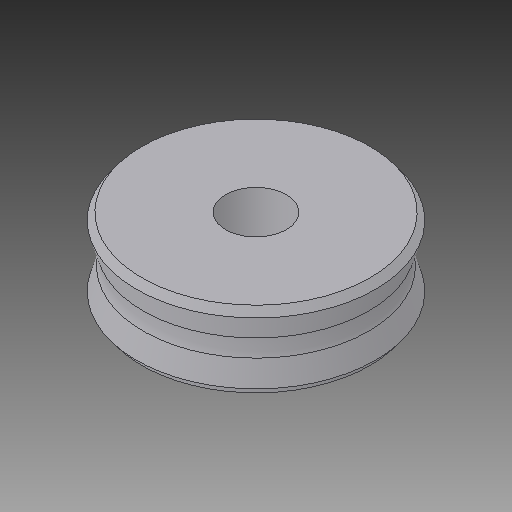
# Autodesk Inventor part: Roulement a bille 634ZZ
Saved by Autodesk Inventor 2017 (Build 210142000, 142)
## iProperties
Company: FABLAB Frenchmakers
Part Number: Roulement a bille 634ZZ
Material: ----------
Document SubType Name: Modeling
Designer: FABLAB Frenchmakers
Density: 7.86 g/cm^3
Appearance: Métal - Acier
Mass: 6.61052 g
Surface Area: 6.47649 cm^2
Volume: 0.841033 cm^3
Project: 1420 Vauban 3D XL
Catalog Web Link: http://frenchmakers.com/
Stock Number: 1420-05-17
Autodesk Inventor part; units mm, degrees
ref_plane "YZ Plane" through (0, 0, 0) normal (1, 0, 0) x (0, 1, 0)
ref_plane "XZ Plane" through (0, 0, 0) normal (0, 1, 0) x (-1, 0, 0)
ref_plane "XY Plane" through (0, 0, 0) normal (0, 0, 1) x (1, 0, 0)
sketch "Esquisse1" plane through (0, 0, 0) normal (0, 0, 1) x (1, 0, 0)
  line L0 (0, 0) -> (0, 2.5152)
  line L1 (2, -2.5) -> (2, 2.5)
  line L2 (2, 2.5) -> (8, 2.5)
  line L3 (8, 2.5) -> (7.4224, 0.5747)
  line L4 (7.4224, -0.5747) -> (8, -2.5)
  line L5 (8, -2.5) -> (2, -2.5)
  arc A0 (7.4224, 0.5747) -> (7.4224, -0.5747) centre (9.3381, 0) ccw
  point P0 (7.25, 0)
  dimension "d0" = 4
  dimension "d1" = 5
  dimension "d2" = 2.5
  dimension "d3" = 16
  dimension "d4" = 14.5
  dimension "d5" = 2
  constraints: 12 end point, 2 point on circle, 2 point on line, 2 tangent, 2 vertical, 1 centre point, 1 horizontal, 1 horizontal alignment, 1 parallel, 1 vertical alignment
  measures "d0" diameter of L1 L0
  measures "d1" distance between parallel lines of L5 L2
  measures "d2" distance from line of L0.start L2
  measures "d3" diameter of L2.end L0
  measures "d4" diameter of point (7.25, 0) L0
  measures "d5" radius of A0
revolve "Révolution1" add sketch "Esquisse1" angle 360 about axis through (0, 0, 0) along (0, 1, 0)
chamfer "Chanfrein1" distance 0.5 angle 45 2 edges at (-8, 2.5, 0) (-8, -2.5, 0)
equation "\"d2\" = 0.5 * d1"
